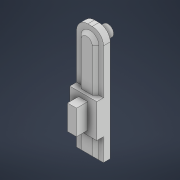
# Autodesk Inventor part: wheel connector
Saved by Autodesk Inventor 2022 (Build 260153000, 153)
## iProperties
Created: 2021-12-22
Part Number: wheel connector
Material: Generic
Document SubType Name: Modeling
Designer: MatusBarany
Density: 1 g/cm^3
Appearance: Default
Author: MatusBarany
Autodesk Inventor part; units mm, degrees
ref_plane "YZ Plane" through (0, 0, 0) normal (1, 0, 0) x (0, 1, 0)
ref_plane "XZ Plane" through (0, 0, 0) normal (0, 1, 0) x (-1, 0, 0)
ref_plane "XY Plane" through (0, 0, 0) normal (0, 0, 1) x (1, 0, 0)
sketch "Sketch1" plane through (0, 0, 0) normal (0, 0, 1) x (1, 0, 0)
  line L0 (-9.9011, 30.8282) -> (2.0989, 30.8282)
  line L1 (2.0989, 30.8282) -> (2.0989, -19.1718)
  line L2 (2.0989, -19.1718) -> (-9.9011, -19.1718)
  line L3 (-9.9011, -19.1718) -> (-9.9011, 30.8282)
  point P0 (0, 0)
  dimension "d0" = 50
  dimension "d1" = 12
  constraints: 8 end point, 2 parallel, 1 horizontal, 1 perpendicular
  measures "d0" distance of L0.end L1.end
  measures "d1" distance of L1.end L2.end
extrude "Extrusion1" add sketch "Sketch1" along normal blind 3
sketch "Sketch2" plane through (0, 0, 0) normal (0, 0, -1) x (-1, 0, 0)
  line L0 (-2.0989, -19.1718) -> (-2.0989, 30.8282) projected
  line L1 (9.9011, -19.1718) -> (-2.0989, -19.1718) projected
  line L2 (-2.0989, -11.1718) -> (9.9011, -11.1718)
  line L3 (9.9011, -11.1718) -> (9.9011, -19.1718)
  line L4 (9.9011, -19.1718) -> (-2.0989, -19.1718)
  line L5 (-2.0989, -19.1718) -> (-2.0989, -11.1718)
  line L6 (-1.0989, -12.1718) -> (8.9011, -12.1718)
  line L7 (8.9011, -12.1718) -> (8.9011, -18.1718)
  line L8 (8.9011, -18.1718) -> (-1.0989, -18.1718)
  line L9 (-1.0989, -18.1718) -> (-1.0989, -12.1718)
  point P0 (0, 0)
  dimension "d1" = 12
  dimension "d4" = 8
  dimension "d5" = 10
  dimension "d6" = 6
  dimension "d7" = 1
  dimension "d8" = 1
  dimension "d9" = 12
  constraints: 16 end point, 4 parallel, 2 horizontal, 2 perpendicular, 1 point on line
  measures "d4" distance between parallel lines of L1 L2
  measures "d5" distance of L6.start L6.end
  measures "d6" distance of L6.end L7.end
  measures "d7" distance between parallel lines of L3 L7
  measures "d8" distance between parallel lines of L2 L6
  measures "d9" distance of L2.start L2.end
extrude "Extrusion2" cut sketch "Sketch2" against normal blind 1 contours L6 L7 L8 L9
sketch "Sketch3" plane through (0, 0, 0) normal (0, 0, -1) x (-1, 0, 0)
  line L0 (-2.0989, -19.1718) -> (-2.0989, 30.8282) projected
  line L1 (-2.0989, 30.8282) -> (9.9011, 30.8282) projected
  line L2 (9.9011, 30.8282) -> (9.9011, -19.1718) projected
  circle A0 centre (3.9011, 24.8282) radius 2.5
  line L3 (-2.0989, 30.8282) -> (9.9011, 30.8282)
  line L4 (9.9011, 30.8282) -> (9.9011, 18.8282)
  line L5 (9.9011, 18.8282) -> (-2.0989, 18.8282)
  line L6 (-2.0989, 18.8282) -> (-2.0989, 30.8282)
  point P0 (0, 0)
  dimension "d12" = 5
  dimension "d13" = 6
  dimension "d14" = 12
  dimension "d15" = 12
  dimension "d16" = 6
  constraints: 8 end point, 2 parallel, 1 centre point, 1 horizontal, 1 perpendicular, 1 point on line
  measures "d12" diameter of A0
  measures "d13" distance from line of L0 A0.centre
  measures "d14" distance of L0.end L1.end
  measures "d15" distance between parallel lines of L1 L5
  measures "d16" distance from line of L1 A0.centre
extrude "Extrusion3" add sketch "Sketch3" along normal blind 5 contours A0
fillet "Fillet1" radius 1 1 edges at (-1.4011, 24.8282, 0)
sketch "Sketch4" plane through (0, 0, 3) normal (0, 0, 1) x (1, 0, 0)
  line L0 (2.0989, -19.1718) -> (2.0989, 30.8282) projected
  line L1 (-9.9011, 5.8282) -> (2.0989, 5.8282)
  line L2 (2.0989, 5.8282) -> (2.0989, -9.1718)
  line L3 (2.0989, -9.1718) -> (-9.9011, -9.1718)
  line L4 (-9.9011, -9.1718) -> (-9.9011, 5.8282)
  line L5 (-9.9011, 30.8282) -> (-9.9011, -19.1718) projected
  line L6 (-9.9011, -19.1718) -> (2.0989, -19.1718) projected
  line L7 (2.0989, -19.1718) -> (2.0989, 30.8282) projected
  line L8 (2.0989, 30.8282) -> (-9.9011, 30.8282) projected
  line L9 (-9.9011, 30.8282) -> (-9.9011, -19.1718) projected
  point P0 (0, 0)
  point P1 (2.0989, 5.8282)
  dimension "d20" = 15
  dimension "d21" = 10
  constraints: 8 end point, 2 parallel, 1 horizontal, 1 midpoint, 1 perpendicular, 1 point on line
  measures "d20" distance between parallel lines of L1 L3
  measures "d21" distance between parallel lines of L3 L6
extrude "Extrusion4" add sketch "Sketch4" along normal blind 3 contours L3 L4 L1 L0
sketch "Sketch5" plane through (0, 0, 6) normal (0, 0, 1) x (1, 0, 0)
  line L0 (-5.9011, 3.8282) -> (-1.9011, 3.8282)
  line L1 (-1.9011, 3.8282) -> (-1.9011, -7.1718)
  line L2 (-1.9011, -7.1718) -> (-5.9011, -7.1718)
  line L3 (-5.9011, -7.1718) -> (-5.9011, 3.8282)
  line L4 (-9.9011, -9.1718) -> (2.0989, -9.1718) projected
  line L5 (2.0989, -9.1718) -> (2.0989, 5.8282) projected
  line L6 (2.0989, 5.8282) -> (-9.9011, 5.8282) projected
  line L7 (-9.9011, 5.8282) -> (-9.9011, -9.1718) projected
  point P0 (0, 0)
  dimension "d24" = 12
  dimension "d25" = 15
  dimension "d26" = 4
  dimension "d27" = 11
  dimension "d28" = 4
  dimension "d29" = 2
  constraints: 8 end point, 2 parallel, 1 horizontal, 1 perpendicular
  measures "d24" distance of L5.end L6.end
  measures "d25" distance of L4.end L5.end
  measures "d26" distance of L0.start L0.end
  measures "d27" distance of L0.end L1.end
  measures "d28" distance between parallel lines of L5 L1
  measures "d29" distance between parallel lines of L6 L0
extrude "Extrusion5" add sketch "Sketch5" along normal blind 5 contours L0 L1 L2 L3
fillet "Fillet2" radius 5 2 edges at (-9.9011, 30.8282, 1.5) (2.0989, 30.8282, 1.5)
sketch "Sketch6" plane through (0, 0, 3) normal (0, 0, 1) x (1, 0, 0)
  circle A0 centre (-3.9011, 24.8282) radius 2.5 projected
  line L0 (-6.4011, 24.8282) -> (-1.4011, 24.8282)
  line L1 (-1.4011, 24.8282) -> (-1.4011, 5.8282)
  line L2 (-1.4011, 5.8282) -> (-6.4011, 5.8282)
  line L3 (-6.4011, 5.8282) -> (-6.4011, 24.8282)
  line L4 (2.0989, 5.8282) -> (-9.9011, 5.8282) projected
  line L5 (2.0989, -9.1718) -> (-9.9011, -9.1718) projected
  line L6 (-6.4011, -9.1718) -> (-1.4011, -9.1718)
  line L7 (-1.4011, -9.1718) -> (-1.4011, -19.1718)
  line L8 (-1.4011, -19.1718) -> (-6.4011, -19.1718)
  line L9 (-6.4011, -19.1718) -> (-6.4011, -9.1718)
  line L10 (-9.9011, -19.1718) -> (2.0989, -19.1718) projected
  point P0 (0, 0)
  point P1 (-1.4011, -9.1718)
  dimension "d38" = 5
  dimension "d39" = 5
  constraints: 16 end point, 4 parallel, 3 collinear, 2 horizontal, 2 perpendicular, 2 vertical, 1 point on line, 2 other
  measures "d38" distance between parallel lines of L1 L3
  measures "d39" distance between parallel lines of L9 L7
extrude "Extrusion6" add sketch "Sketch6" along normal blind 1.5
chamfer "Chamfer1" distance 1.5 angle 45 6 edges at (-1.4011, 15.3282, 3) (-3.9011, 27.3282, 3) (-6.4011, 15.3282, 3) (-6.4011, -14.1718, 3) (-1.4011, -14.1718, 3) (-3.9011, -19.1718, 4.5)
equation "\"d7\" = -0.5 * d5 + 0.5 * d9"
equation "\"d8\" = -0.5 * d6 + 0.5 * d4"
equation "\"d13\" = 0.5 * d14"
equation "\"d15\" = d14"
equation "\"d16\" = 0.5 * d14"
equation "\"d26\" = 0.333333 * d24"
equation "\"d28\" = -0.5 * d26 + 0.5 * d24"
equation "\"d39\" = d38"
body "Solid1"
